Autodesk Inventor part; units mm, degrees
(part 2 of 2)
  line L756 (-570.9199, 958.9434) -> (-599.5987, 917.9858)
  line L757 (-652.8436, 955.2683) -> (-693.8012, 983.9471)
  line L758 (-693.8012, 983.9471) -> (-665.1223, 1024.9047)
  line L759 (-665.1223, 1024.9047) -> (-624.1647, 996.2259)
  line L760 (-624.1647, 996.2259) -> (-652.8436, 955.2683)
  line L761 (-706.0884, 992.5508) -> (-747.0461, 1021.2296)
  line L762 (-747.0461, 1021.2296) -> (-718.3672, 1062.1872)
  line L763 (-718.3672, 1062.1872) -> (-677.4096, 1033.5084)
  line L764 (-677.4096, 1033.5084) -> (-706.0884, 992.5508)
  line L765 (-759.3333, 1029.8332) -> (-800.2909, 1058.512)
  line L766 (-800.2909, 1058.512) -> (-771.6121, 1099.4696)
  line L767 (-771.6121, 1099.4696) -> (-730.6545, 1070.7908)
  line L768 (-730.6545, 1070.7908) -> (-759.3333, 1029.8332)
  line L769 (-812.5782, 1067.1157) -> (-853.5358, 1095.7945)
  line L770 (-853.5358, 1095.7945) -> (-824.857, 1136.7521)
  line L771 (-824.857, 1136.7521) -> (-783.8994, 1108.0733)
  line L772 (-783.8994, 1108.0733) -> (-812.5782, 1067.1157)
  line L773 (-865.8231, 1104.3982) -> (-906.7807, 1133.077)
  line L774 (-906.7807, 1133.077) -> (-878.1019, 1174.0346)
  line L775 (-878.1019, 1174.0346) -> (-837.1443, 1145.3558)
  line L776 (-837.1443, 1145.3558) -> (-865.8231, 1104.3982)
  line L777 (-919.068, 1141.6806) -> (-960.0256, 1170.3595)
  line L778 (-960.0256, 1170.3595) -> (-931.3468, 1211.3171)
  line L779 (-931.3468, 1211.3171) -> (-890.3892, 1182.6382)
  line L780 (-890.3892, 1182.6382) -> (-919.068, 1141.6806)
  line L781 (-210.9221, 566.4812) -> (-251.8797, 595.16)
  line L782 (-251.8797, 595.16) -> (-223.2009, 636.1176)
  line L783 (-223.2009, 636.1176) -> (-182.2433, 607.4388)
  line L784 (-182.2433, 607.4388) -> (-210.9221, 566.4812)
  line L785 (-264.167, 603.7637) -> (-305.1246, 632.4425)
  line L786 (-305.1246, 632.4425) -> (-276.4458, 673.4001)
  line L787 (-276.4458, 673.4001) -> (-235.4881, 644.7213)
  line L788 (-235.4881, 644.7213) -> (-264.167, 603.7637)
  line L789 (-317.4119, 641.0461) -> (-358.3695, 669.7249)
  line L790 (-358.3695, 669.7249) -> (-329.6906, 710.6826)
  line L791 (-329.6906, 710.6826) -> (-288.733, 682.0037)
  line L792 (-288.733, 682.0037) -> (-317.4119, 641.0461)
  line L793 (-370.6567, 678.3286) -> (-411.6143, 707.0074)
  line L794 (-411.6143, 707.0074) -> (-382.9355, 747.965)
  line L795 (-382.9355, 747.965) -> (-341.9779, 719.2862)
  line L796 (-341.9779, 719.2862) -> (-370.6567, 678.3286)
  line L797 (-423.9016, 715.6111) -> (-464.8592, 744.2899)
  line L798 (-464.8592, 744.2899) -> (-436.1804, 785.2475)
  line L799 (-436.1804, 785.2475) -> (-395.2228, 756.5687)
  line L800 (-395.2228, 756.5687) -> (-423.9016, 715.6111)
  line L801 (-477.1465, 752.8935) -> (-518.1041, 781.5724)
  line L802 (-518.1041, 781.5724) -> (-489.4253, 822.53)
  line L803 (-489.4253, 822.53) -> (-448.4677, 793.8511)
  line L804 (-448.4677, 793.8511) -> (-477.1465, 752.8935)
  line L805 (-530.3914, 790.176) -> (-571.349, 818.8548)
  line L806 (-571.349, 818.8548) -> (-542.6702, 859.8124)
  line L807 (-542.6702, 859.8124) -> (-501.7126, 831.1336)
  line L808 (-501.7126, 831.1336) -> (-530.3914, 790.176)
  line L809 (-583.6363, 827.4585) -> (-624.5939, 856.1373)
  line L810 (-624.5939, 856.1373) -> (-595.915, 897.0949)
  line L811 (-595.915, 897.0949) -> (-554.9574, 868.4161)
  line L812 (-554.9574, 868.4161) -> (-583.6363, 827.4585)
  line L813 (-636.8812, 864.7409) -> (-677.8388, 893.4198)
  line L814 (-677.8388, 893.4198) -> (-649.1599, 934.3774)
  line L815 (-649.1599, 934.3774) -> (-608.2023, 905.6985)
  line L816 (-608.2023, 905.6985) -> (-636.8812, 864.7409)
  line L817 (-690.126, 902.0234) -> (-731.0836, 930.7022)
  line L818 (-731.0836, 930.7022) -> (-702.4048, 971.6598)
  line L819 (-702.4048, 971.6598) -> (-661.4472, 942.981)
  line L820 (-661.4472, 942.981) -> (-690.126, 902.0234)
  line L821 (-743.3709, 939.3059) -> (-784.3285, 967.9847)
  line L822 (-784.3285, 967.9847) -> (-755.6497, 1008.9423)
  line L823 (-755.6497, 1008.9423) -> (-714.6921, 980.2635)
  line L824 (-714.6921, 980.2635) -> (-743.3709, 939.3059)
  line L825 (-796.6158, 976.5883) -> (-837.5734, 1005.2672)
  line L826 (-837.5734, 1005.2672) -> (-808.8946, 1046.2248)
  line L827 (-808.8946, 1046.2248) -> (-767.937, 1017.5459)
  line L828 (-767.937, 1017.5459) -> (-796.6158, 976.5883)
  line L829 (-849.8607, 1013.8708) -> (-890.8183, 1042.5496)
  line L830 (-890.8183, 1042.5496) -> (-862.1395, 1083.5072)
  line L831 (-862.1395, 1083.5072) -> (-821.1819, 1054.8284)
  line L832 (-821.1819, 1054.8284) -> (-849.8607, 1013.8708)
  line L833 (-903.1056, 1051.1533) -> (-944.0632, 1079.8321)
  line L834 (-944.0632, 1079.8321) -> (-915.3843, 1120.7897)
  line L835 (-915.3843, 1120.7897) -> (-874.4267, 1092.1109)
  line L836 (-874.4267, 1092.1109) -> (-903.1056, 1051.1533)
  line L837 (-956.3504, 1088.4357) -> (-997.3081, 1117.1146)
  line L838 (-997.3081, 1117.1146) -> (-968.6292, 1158.0722)
  line L839 (-968.6292, 1158.0722) -> (-927.6716, 1129.3933)
  line L840 (-927.6716, 1129.3933) -> (-956.3504, 1088.4357)
  line L841 (-248.2046, 513.2363) -> (-289.1622, 541.9151)
  line L842 (-289.1622, 541.9151) -> (-260.4833, 582.8727)
  line L843 (-260.4833, 582.8727) -> (-219.5257, 554.1939)
  line L844 (-219.5257, 554.1939) -> (-248.2046, 513.2363)
  line L845 (-301.4494, 550.5188) -> (-342.407, 579.1976)
  line L846 (-342.407, 579.1976) -> (-313.7282, 620.1552)
  line L847 (-313.7282, 620.1552) -> (-272.7706, 591.4764)
  line L848 (-272.7706, 591.4764) -> (-301.4494, 550.5188)
  line L849 (-354.6943, 587.8012) -> (-395.6519, 616.4801)
  line L850 (-395.6519, 616.4801) -> (-366.9731, 657.4377)
  line L851 (-366.9731, 657.4377) -> (-326.0155, 628.7588)
  line L852 (-326.0155, 628.7588) -> (-354.6943, 587.8012)
  line L853 (-407.9392, 625.0837) -> (-448.8968, 653.7625)
  line L854 (-448.8968, 653.7625) -> (-420.218, 694.7201)
  line L855 (-420.218, 694.7201) -> (-379.2604, 666.0413)
  line L856 (-379.2604, 666.0413) -> (-407.9392, 625.0837)
  line L857 (-461.1841, 662.3662) -> (-502.1417, 691.045)
  line L858 (-502.1417, 691.045) -> (-473.4629, 732.0026)
  line L859 (-473.4629, 732.0026) -> (-432.5053, 703.3238)
  line L860 (-432.5053, 703.3238) -> (-461.1841, 662.3662)
  line L861 (-514.429, 699.6486) -> (-555.3866, 728.3275)
  line L862 (-555.3866, 728.3275) -> (-526.7078, 769.2851)
  line L863 (-526.7078, 769.2851) -> (-485.7501, 740.6063)
  line L864 (-485.7501, 740.6063) -> (-514.429, 699.6486)
  line L865 (-567.6739, 736.9311) -> (-608.6315, 765.6099)
  line L866 (-608.6315, 765.6099) -> (-579.9526, 806.5675)
  line L867 (-579.9526, 806.5675) -> (-538.995, 777.8887)
  line L868 (-538.995, 777.8887) -> (-567.6739, 736.9311)
  line L869 (-620.9187, 774.2136) -> (-661.8763, 802.8924)
  line L870 (-661.8763, 802.8924) -> (-633.1975, 843.85)
  line L871 (-633.1975, 843.85) -> (-592.2399, 815.1712)
  line L872 (-592.2399, 815.1712) -> (-620.9187, 774.2136)
  line L873 (-674.1636, 811.4961) -> (-715.1212, 840.1749)
  line L874 (-715.1212, 840.1749) -> (-686.4424, 881.1325)
  line L875 (-686.4424, 881.1325) -> (-645.4848, 852.4537)
  line L876 (-645.4848, 852.4537) -> (-674.1636, 811.4961)
  line L877 (-727.4085, 848.7785) -> (-768.3661, 877.4573)
  line L878 (-768.3661, 877.4573) -> (-739.6873, 918.4149)
  line L879 (-739.6873, 918.4149) -> (-698.7297, 889.7361)
  line L880 (-698.7297, 889.7361) -> (-727.4085, 848.7785)
  line L881 (-780.6534, 886.061) -> (-821.611, 914.7398)
  line L882 (-821.611, 914.7398) -> (-792.9322, 955.6974)
  line L883 (-792.9322, 955.6974) -> (-751.9746, 927.0186)
  line L884 (-751.9746, 927.0186) -> (-780.6534, 886.061)
  line L885 (-833.8983, 923.3435) -> (-874.8559, 952.0223)
  line L886 (-874.8559, 952.0223) -> (-846.177, 992.9799)
  line L887 (-846.177, 992.9799) -> (-805.2194, 964.3011)
  line L888 (-805.2194, 964.3011) -> (-833.8983, 923.3435)
  line L889 (-887.1432, 960.6259) -> (-928.1008, 989.3047)
  line L890 (-928.1008, 989.3047) -> (-899.4219, 1030.2624)
  line L891 (-899.4219, 1030.2624) -> (-858.4643, 1001.5835)
  line L892 (-858.4643, 1001.5835) -> (-887.1432, 960.6259)
  line L893 (-940.388, 997.9084) -> (-981.3456, 1026.5872)
  line L894 (-981.3456, 1026.5872) -> (-952.6668, 1067.5448)
  line L895 (-952.6668, 1067.5448) -> (-911.7092, 1038.866)
  line L896 (-911.7092, 1038.866) -> (-940.388, 997.9084)
  line L897 (-993.6329, 1035.1909) -> (-1034.5905, 1063.8697)
  line L898 (-1034.5905, 1063.8697) -> (-1005.9117, 1104.8273)
  line L899 (-1005.9117, 1104.8273) -> (-964.9541, 1076.1485)
  line L900 (-964.9541, 1076.1485) -> (-993.6329, 1035.1909)
  line L901 (-360, 1485) -> (-360, 885) projected
  line L902 (-360, 885) -> (-660, 885) projected
  line L903 (-660, 885) -> (-660, 1485) projected
  line L904 (-660, 1485) -> (-360, 1485) projected
  line L905 (-320, 1485) -> (-20, 1485) projected
  line L906 (-20, 1485) -> (-20, 885) projected
  line L907 (-20, 885) -> (-320, 885) projected
  line L908 (-320, 885) -> (-320, 1485) projected
  line L909 (0, 840) -> (0, 1515) projected
  line L910 (0, 1515) -> (-715, 1515) projected
  line L911 (-715, 1515) -> (-715, 840) projected
  line L912 (0, 840) -> (-715, 840) projected
  point P0 (0, 0)
  point P1 (-20, 1446.039)
  point P2 (-20, 1464.3506)
  point P3 (-25.5588, 1485)
  point P4 (-43.8704, 1485)
  point P5 (-49.4904, 1485)
  point P6 (-75.6421, 1485)
  point P7 (-104.9091, 1485)
  point P8 (-123.2207, 1485)
  point P9 (-162.8144, 1485)
  point P10 (-202.5711, 1485)
  point P11 (-263.6098, 1485)
  point P12 (-302.2901, 1485)
  point P13 (-320, 1436.3618)
  point P14 (-320, 1404.4665)
  point P15 (-320, 1357.0115)
  point P16 (-320, 1338.6999)
  point P17 (-320, 1317.2941)
  point P18 (-320, 1291.1424)
  point P19 (-320, 1277.6612)
  point P20 (-320, 1259.3495)
  point P21 (-320, 1203.9701)
  point P22 (-320, 1177.8184)
  point P23 (-320, 1118.9605)
  point P24 (-320, 1100.6488)
  point P25 (-320, 1090.646)
  point P26 (-320, 1064.4943)
  point P27 (-320, 1039.6101)
  point P28 (-320, 1021.2985)
  point P29 (-320, 977.322)
  point P30 (-320, 941.9481)
  point P31 (-305.2942, 885)
  point P32 (-286.9826, 885)
  point P33 (-238.6696, 885)
  point P34 (-207.6322, 885)
  point P35 (-146.5935, 885)
  point P36 (-128.2819, 885)
  point P37 (-125.3456, 885)
  point P38 (-99.1939, 885)
  point P39 (-67.2432, 885)
  point P40 (-48.9315, 885)
  point P41 (-20, 890.5866)
  point P42 (-20, 908.8982)
  point P43 (-20, 926.3185)
  point P44 (-20, 952.4702)
  point P45 (-20, 969.9369)
  point P46 (-20, 988.2485)
  point P47 (-20, 1039.6426)
  point P48 (-20, 1067.5989)
  point P49 (-20, 1128.6376)
  point P50 (-20, 1146.9492)
  point P51 (-20, 1152.9666)
  point P52 (-20, 1179.1183)
  point P53 (-20, 1207.988)
  point P54 (-20, 1226.2996)
  point P55 (-20, 1266.2907)
  point P56 (-20, 1305.6499)
  point P57 (-20, 1366.6887)
  point P58 (-20, 1405.7664)
  point P59 (-360, 1446.0585)
  point P60 (-361.2718, 1485)
  point P61 (-389.4625, 1485)
  point P62 (-415.6142, 1485)
  point P63 (-422.3105, 1485)
  point P64 (-440.6221, 1485)
  point P65 (-501.6609, 1485)
  point P66 (-528.9382, 1485)
  point P67 (-581.0112, 1485)
  point P68 (-599.3228, 1485)
  point P69 (-616.1106, 1485)
  point P70 (-642.2623, 1485)
  point P71 (-660, 1436.3814)
  point P72 (-660, 1418.0697)
  point P73 (-660, 1398.344)
  point P74 (-660, 1372.1923)
  point P75 (-660, 1357.031)
  point P76 (-660, 1338.7194)
  point P77 (-660, 1285.02)
  point P78 (-660, 1258.8683)
  point P79 (-660, 1198.3303)
  point P80 (-660, 1180.0187)
  point P81 (-660, 1171.6959)
  point P82 (-660, 1145.5442)
  point P83 (-660, 1118.98)
  point P84 (-660, 1100.6684)
  point P85 (-660, 1058.3719)
  point P86 (-660, 1021.318)
  point P87 (-660, 960.2793)
  point P88 (-660, 918.8961)
  point P89 (-622.6956, 885)
  point P90 (-604.384, 885)
  point P91 (-578.6418, 885)
  point P92 (-552.4901, 885)
  point P93 (-543.3453, 885)
  point P94 (-525.0336, 885)
  point P95 (-465.3177, 885)
  point P96 (-439.166, 885)
  point P97 (-384.6446, 885)
  point P98 (-366.3329, 885)
  point P99 (-360, 890.6061)
  point P100 (-360, 920.1961)
  point P101 (-360, 969.9564)
  point P102 (-360, 988.2681)
  point P103 (-360, 1007.3684)
  point P104 (-360, 1033.5201)
  point P105 (-360, 1049.3068)
  point P106 (-360, 1067.6184)
  point P107 (-360, 1120.6925)
  point P108 (-360, 1146.9688)
  point P109 (-360, 1208.0075)
  point P110 (-360, 1226.3191)
  point P111 (-360, 1234.0165)
  point P112 (-360, 1260.1682)
  point P113 (-360, 1287.3578)
  point P114 (-360, 1305.6695)
  point P115 (-360, 1347.3405)
  point P116 (-360, 1385.0198)
  dimension "d68" = 50
  dimension "d69" = 50
  dimension "d70" = 35
  dimension "d73" = 65
  dimension "d76" = 65
  constraints: 1800 end point, 2 collinear, 2 parallel, 1 perpendicular, 1796 other
  measures "d68" distance of L0.start L0.end
  measures "d69" distance of L0.end L1.end
  measures "d70" angle of L4 L0
  measures "d73" distance of L0.start L5.start
  measures "d76" distance of L0.start L61.start
extrude "Extrusion5" add sketch "Sketch3" along normal blind 2 and the other way blind 20 contours L4 L684 L683 L682 L681 L747 L746 L752 L751 L750 L749 L811 L810 L816 L815 L814 L903 L757 L760 L759 L704 L703 L641 L644 L643 L642 L648 L647 L585 L588 L587 L586 L532 L531 L469 L472 L471 L470 L476 L475 L413 L416 L415 L904 L353 L356 L350 L349 L352 L351 L286 L285 L288 L282 L281 L284 L283 L221 L224 L901 L279 L278 L277 L334 L333 L395 L394 L393 L396 L390 L389 L451 L450 L449 L506 L505 L567 L566 L565 L568 L562 L561 L623 L622 L621 L624 L679 L678 | L564 L563 L908 L501 L504 L503 L502 L508 L507 L445 L448 L447 L446 L392 L391 L329 L332 L331 L330 L336 L335 L273 L276 L275 L274 L217 L220 L219 L905 L154 L153 L156 L89 L92 L86 L85 L88 L87 L25 L28 L22 L21 L906 L83 L82 L81 L84 L139 L138 L137 L194 L193 L255 L254 L253 L256 L250 L249 L311 L310 L309 L366 L365 L427 L426 L425 L428 L422 L421 L483 L482 L907 L488 L487 L486 L485 L547 L546 L552 L551 L550 L615 L614 L620 L619
chamfer "Chamfer1" distance 30 angle 45 2 edges at (-372.5, 70, -840) (-797.5, 70, -787.5)
chamfer "Chamfer2" distance 30 angle 45 2 edges at (-787.5, 40, -490) (-810, 40, -25)
sketch "Sketch5" plane through (-715, 0, -1515) normal (-1, 0, 0) x (0, 0, 1)
  line L0 (0, 0) -> (0, 40) projected
  line L1 (0, 40) -> (-50, 8)
  line L2 (-50, 8) -> (-50, 0)
  line L3 (-50, 0) -> (0, 0)
  point P0 (1515, 0)
  dimension "d89" = 50
  dimension "d90" = 8
  constraints: 6 end point, 1 parallel, 1 perpendicular
  measures "d89" distance between parallel lines of L0 L2
  measures "d90" distance of L1.end L2.end
extrude "Extrusion6" add sketch "Sketch5" against normal up to surface (715 mm away)
sketch "Sketch6" plane through (-850, 0, 0) normal (0, 0, 1) x (1, 0, 0)
  line L0 (0, 20) -> (10, 20)
  line L1 (10, 20) -> (10, 50)
  line L2 (10, 50) -> (0, 50)
  line L3 (0, 50) -> (0, 20)
  line L4 (0, 0) -> (0, 70) projected
  line L5 (0, 0) -> (85, 0) projected
  circle A0 centre (5, 50) radius 3
  circle A1 centre (5, 20) radius 3
  point P0 (850, 0)
  point P1 (8, 50)
  point P2 (2, 50)
  point P3 (2, 20)
  point P4 (8, 20)
  dimension "d93" = 10
  dimension "d94" = 20
  dimension "d95" = 30
  dimension "d96" = 6
  dimension "d97" = 6
  constraints: 8 end point, 2 centre point, 2 midpoint, 2 parallel, 1 collinear, 1 horizontal, 1 perpendicular
  measures "d93" distance between parallel lines of L3 L1
  measures "d94" distance between parallel lines of L5 L0
  measures "d95" distance between parallel lines of L0 L2
  measures "d96" diameter of A0
  measures "d97" diameter of A1
extrude "Extrusion7" cut sketch "Sketch6" against normal through all contours A1 L0 L3 L2 A0 L1
mirror "Mirror1" about plane through (0, 0, 0) normal (1, 0, 0) of "Extrusion1", "Extrusion3", "Extrusion4", "Extrusion5", "Chamfer1", "Chamfer2", "Extrusion6", "Extrusion7"
equation "\"d65\" = d60"
body "Solid1"
